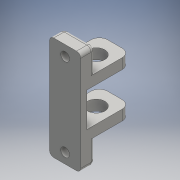
# Autodesk Inventor part: support_roue_bascule
Saved by Autodesk Inventor 2016 (Build 200138000, 138)
## iProperties
Created: 2017-05-12
Part Number: support_roue_bascule
Material: Générique
Document SubType Name: Modeling
Designer: Galileo
Density: 1 g/cm^3
Appearance: Par défaut
Author: Galileo
Autodesk Inventor part; units mm, degrees
ref_plane "YZ Plane" through (0, 0, 0) normal (1, 0, 0) x (0, 1, 0)
ref_plane "XZ Plane" through (0, 0, 0) normal (0, 1, 0) x (-1, 0, 0)
ref_plane "XY Plane" through (0, 0, 0) normal (0, 0, 1) x (1, 0, 0)
sketch "Esquisse1" plane through (0, 0, 0) normal (0, 1, 0) x (-1, 0, 0)
  line L0 (0, 0) -> (15, 0)
  line L1 (15, 0) -> (15, -50)
  line L2 (15, -50) -> (0, -50)
  line L3 (0, -50) -> (0, 0)
  dimension "d0" = 50
  dimension "d1" = 15
  constraints: 8 end point, 2 parallel, 1 horizontal, 1 perpendicular
  measures "d0" distance of L2.end L0.start
  measures "d1" distance of L0.start L0.end
extrude "Extrusion1" add sketch "Esquisse1" along normal blind 3
sketch "Esquisse2" plane through (0, 3, 0) normal (0, 1, 0) x (1, 0, 0)
  line L0 (-15, 50) -> (-15, 0) projected
  line L1 (-15, 11.75) -> (0, 11.75)
  line L2 (0, 11.75) -> (0, 38.25)
  line L3 (0, 38.25) -> (-15, 38.25)
  line L4 (-15, 38.25) -> (-15, 11.75)
  line L5 (-15, 0) -> (0, 0) projected
  line L6 (0, 50) -> (-15, 50) projected
  line L7 (-15, 11.75) -> (0, 11.75)
  line L8 (0, 11.75) -> (0, 16.75)
  line L9 (0, 16.75) -> (-15, 16.75)
  line L10 (-15, 16.75) -> (-15, 11.75)
  line L11 (-15, 33.25) -> (0, 33.25)
  line L12 (0, 33.25) -> (0, 38.25)
  line L13 (0, 38.25) -> (-15, 38.25)
  line L14 (-15, 38.25) -> (-15, 33.25)
  dimension "d4" = 15
  dimension "d5" = 11.75
  dimension "d6" = 11.75
  dimension "d7" = 5
  dimension "d8" = 5
  constraints: 24 end point, 6 parallel, 3 horizontal, 3 perpendicular, 3 point on line
  measures "d4" distance of L2.end L3.end
  measures "d5" distance between parallel lines of L5 L1
  measures "d6" distance between parallel lines of L6 L3
  measures "d7" distance between parallel lines of L1 L9
  measures "d8" distance between parallel lines of L13 L11
extrude "Extrusion2" add sketch "Esquisse2" along normal blind 21 contours L3 L2 L11 L0 | L9 L2 L1 L0
sketch "Esquisse3" plane through (-15, 3, -11.75) normal (0, 0, 1) x (1, 0, 0)
  line L0 (0, 0) -> (15, 0) projected
  line L1 (0, 0) -> (0, 21) projected
  point P0 (15, -3)
  point P1 (7.5, 12)
  dimension "d11" = 12
  dimension "d12" = 7.5
  measures "d11" distance from line of L0 point (7.5, 12)
  measures "d12" distance from line of L1 point (7.5, 12)
hole "Perçage1" at (-7.5, 15, -11.75) direction (0, 0, -1) diameter 8.3 depth 100 tip angle 118
fillet "Congé1" radius 4 1 edges at (0, 24, -14.25)
fillet "Congé2" radius 4 1 edges at (-15, 24, -14.25)
fillet "Congé3" radius 4 1 edges at (-15, 24, -35.75)
fillet "Congé4" radius 4 1 edges at (0, 24, -35.75)
sketch "Esquisse4" plane through (0, 3, 0) normal (0, 1, 0) x (1, 0, 0)
  line L0 (0, 50) -> (0, 0) projected
  line L1 (-15, 0) -> (0, 0)
  line L2 (0, 0) -> (0, 11.75)
  line L3 (0, 11.75) -> (-15, 11.75)
  line L4 (-15, 11.75) -> (-15, 0)
  line L5 (-15, 0) -> (-15, 50) projected
  line L6 (-15, 38.25) -> (0, 38.25) projected
  line L7 (-15, 50) -> (0, 50)
  line L8 (0, 50) -> (0, 38.25)
  line L9 (0, 38.25) -> (-15, 38.25)
  line L10 (-15, 38.25) -> (-15, 50)
  dimension "d24" = 11.75
  dimension "d25" = 15
  constraints: 16 end point, 4 parallel, 2 horizontal, 2 perpendicular, 1 point on line
  measures "d24" distance of L3.end L1.start
  measures "d25" distance of L1.start L1.end
extrude "Extrusion3" add sketch "Esquisse4" along normal blind 4 contours L0 L6 L5 L7 | L0 L1 L4 L3
fillet "Congé5" radius 2 1 edges at (-7.5, 7, 0)
fillet "Congé6" radius 2 1 edges at (-7.5, 7, -50)
fillet "Congé7" radius 2 3 edges at (0, 7, -43.125) (0, 6.4142, -49.4142) (0, 2.5, -50)
fillet "Congé8" radius 2 3 edges at (0, 7, -6.875) (0, 6.4142, -0.5858) (0, 2.5, 0)
fillet "Congé9" radius 2 3 edges at (-15, 7, -6.875) (-15, 6.4142, -0.5858) (-15, 2.5, 0)
fillet "Congé10" radius 2 3 edges at (-15, 7, -43.125) (-15, 6.4142, -49.4142) (-15, 2.5, -50)
sketch "Esquisse5" plane through (0, 7, 0) normal (0, 1, 0) x (1, 0, 0)
  line L0 (-2, 50) -> (-13, 50) projected
  line L1 (0, 38.25) -> (0, 48) projected
  line L2 (0, 2) -> (0, 11.75) projected
  line L3 (-13, 0) -> (-2, 0) projected
  point P0 (0, 0)
  point P1 (-7.5, 45)
  point P2 (-7.5, 5)
  dimension "d34" = 5
  dimension "d35" = 7.5
  dimension "d36" = 7.5
  dimension "d37" = 5
  measures "d34" distance from line of L0 point (-7.5, 45)
  measures "d35" distance from line of L1 point (-7.5, 45)
  measures "d36" distance from line of L2 point (-7.5, 5)
  measures "d37" distance from line of L3 point (-7.5, 5)
hole "Perçage2" at (-7.5, 7, -45) at (-7.5, 7, -5) direction (0, -1, 0) diameter 4.2 depth 100 tip angle 118 countersink diameter 6.5 countersink angle 90
